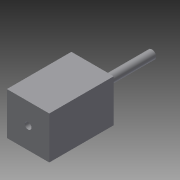
# Autodesk Inventor part: p80 space thing
Saved by Autodesk Inventor 2013 (Build 170138000, 138)
## iProperties
Created: 2013-02-03
Part Number: p80 space thing
Material: Generic
Document SubType Name: Modeling
Designer: Arpan
Density: 1 g/cm^3
Author: Arpan
Autodesk Inventor part; units mm, degrees
ref_plane "YZ Plane" through (0, 0, 0) normal (1, 0, 0) x (0, 1, 0)
ref_plane "XZ Plane" through (0, 0, 0) normal (0, 1, 0) x (-1, 0, 0)
ref_plane "XY Plane" through (0, 0, 0) normal (0, 0, 1) x (1, 0, 0)
sketch "Sketch1" plane through (0, 0, 0) normal (0, 0, 1) x (1, 0, 0)
  line L0 (0, 0) -> (-63.5, 0)
  line L1 (-63.5, 0) -> (-63.5, 63.5)
  line L2 (-63.5, 63.5) -> (0, 63.5)
  line L3 (0, 63.5) -> (0, 0)
  dimension "d0" = 63.5
  dimension "d1" = 63.5
  constraints: 8 end point, 2 parallel, 1 horizontal, 1 perpendicular
  measures "d0" distance of L0.start L0.end
  measures "d1" distance of L0.end L1.end
extrude "Extrusion1" add sketch "Sketch1" along normal blind 96.647
sketch "Sketch2" plane through (0, 0, 0) normal (0, 0, -1) x (-1, 0, 0)
  line L0 (0, 0) -> (63.5, 0) projected
  line L1 (0, 63.5) -> (0, 0) projected
  circle A0 centre (31.75, 31.75) radius 6.35
  dimension "d4" = 12.7
  dimension "d5" = 31.75
  dimension "d6" = 31.75
  constraints: 1 centre point
  measures "d4" diameter of A0
  measures "d5" distance from line of L1 A0.centre
  measures "d6" distance from line of L0 A0.centre
extrude "Extrusion2" add sketch "Sketch2" along normal blind 88.9
sketch "Sketch3" plane through (0, 0, 96.647) normal (0, 0, 1) x (1, 0, 0)
  line L0 (-63.5, 0) -> (0, 0) projected
  line L1 (0, 63.5) -> (-63.5, 63.5) projected
  line L2 (-31.75, 63.5) -> (-31.75, 0)
  circle A0 centre (-31.75, 31.75) radius 5
  dimension "d9" = 63.5
  dimension "d10" = 10
  constraints: 3 midpoint, 2 end point, 1 centre point
  measures "d9" distance of L2.start L2.end
  measures "d10" diameter of A0
extrude "Extrusion3" cut sketch "Sketch3" against normal blind 88.9
body "Solid1"
